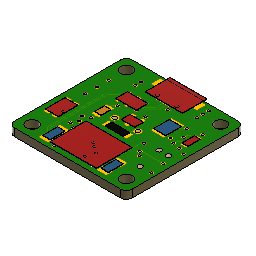
caps-lock-buzzer-v2-v5 (Autodesk Fusion 360 archive; units mm, degrees)
design "caps-lock-buzzer-v2-temp"
part number: 0.1uF 50V
part number: 1uF 16V X5R
part number: PIC16F1459-I/SS
part number: FMMT619TA
part number: 1N4148W-TP
part number: 2.2k
part number: CX-0905C
part number: PRTR5V0U2X
part number: RED
part number: KMR211NGLFS
Autodesk Fusion 360 part; units mm, degrees
sketch "sketch 305" plane through (0, 0, 0) normal (0, 0, 1) x (1, 0, 0)
  line L0 (1.27, 0) -> (24.13, 0)
  arc A0 (24.13, 0) -> (25.4, 1.27) centre (24.13, 1.27) ccw
  line L1 (25.4, 1.27) -> (25.4, 24.13)
  arc A1 (25.4, 24.13) -> (24.13, 25.4) centre (24.13, 24.13) ccw
  line L2 (24.13, 25.4) -> (1.27, 25.4)
  arc A2 (1.27, 25.4) -> (0, 24.13) centre (1.27, 24.13) ccw
  line L3 (0, 24.13) -> (0, 1.27)
  arc A3 (0, 1.27) -> (1.27, 0) centre (1.27, 1.27) ccw
  circle A4 centre (2.54, 2.54) radius 1.27
  circle A5 centre (2.54, 22.86) radius 1.27
  circle A6 centre (22.86, 22.86) radius 1.27
  circle A7 centre (22.86, 2.54) radius 1.27
extrude "Board" add sketch "sketch 305" along normal blind 1.6711 makes body 1 in component "Board"
sketch "sketch 829" plane through (0, 0, 0) normal (0, 0, 1) x (1, 0, 0)
  line L0 (-1.6, -0.8) -> (1.6, -0.8)
  line L1 (1.6, -0.8) -> (1.6, 0.8)
  line L2 (1.6, 0.8) -> (-1.6, 0.8)
  line L3 (-1.6, 0.8) -> (-1.6, -0.8)
extrude "C1206K" add sketch "sketch 829" along normal blind 0.1 separate body makes body 2 in component "C1206K"
sketch "sketch 961" plane through (0, 0, 0) normal (0, 0, 1) x (1, 0, 0)
  line L0 (-1.702, -1.304) -> (1.702, -1.304)
  line L1 (1.702, -1.304) -> (1.702, 1.304)
  line L2 (1.702, 1.304) -> (-1.702, 1.304)
  line L3 (-1.702, 1.304) -> (-1.702, -1.304)
extrude "C1210" add sketch "sketch 961" along normal blind 0.1 separate body makes body 3 in component "C1210"
sketch "sketch 1093" plane through (0, 0, 0) normal (0, 0, 1) x (1, 0, 0)
  line L0 (-4, -2.15) -> (4, -2.15)
  line L1 (4, -2.15) -> (4, 3.15)
  line L2 (4, 3.15) -> (-4, 3.15)
  line L3 (-4, 3.15) -> (-4, -2.15)
extrude "629105136821" add sketch "sketch 1093" along normal blind 0.1 separate body makes body 4 in component "629105136821"
sketch "sketch 1225" plane through (0, 0, 0) normal (0, 0, 1) x (1, 0, 0)
  line L0 (-4.966, -3.861) -> (4.966, -3.861)
  line L1 (4.966, -3.861) -> (4.966, 3.861)
  line L2 (4.966, 3.861) -> (-4.966, 3.861)
  line L3 (-4.966, 3.861) -> (-4.966, -3.861)
extrude "SSOP20_MC" add sketch "sketch 1225" along normal blind 0.1 separate body makes body 5 in component "SSOP20_MC"
sketch "sketch 1357" plane through (0, 0, 0) normal (0, 0, 1) x (1, 0, 0)
  line L0 (-1.422, -0.94) -> (1.473, -0.94)
  line L1 (1.473, -0.94) -> (1.473, 0.94)
  line L2 (1.473, 0.94) -> (-1.422, 0.94)
  line L3 (-1.422, 0.94) -> (-1.422, -0.94)
extrude "SOT-23" add sketch "sketch 1357" along normal blind 0.1 separate body makes body 6 in component "SOT-23"
sketch "sketch 1489" plane through (0, 0, 0) normal (0, 0, 1) x (1, 0, 0)
  line L0 (-1.95, -0.7) -> (1.95, -0.7)
  line L1 (1.95, -0.7) -> (1.95, 0.7)
  line L2 (1.95, 0.7) -> (-1.95, 0.7)
  line L3 (-1.95, 0.7) -> (-1.95, -0.7)
extrude "SOD123" add sketch "sketch 1489" along normal blind 0.1 separate body makes body 7 in component "SOD123"
sketch "sketch 1629" plane through (0, 0, 0) normal (0, 0, 1) x (1, 0, 0)
  line L0 (-1.067, -0.698) -> (1.056, -0.698)
  line L1 (1.056, -0.698) -> (1.056, 0.702)
  line L2 (1.056, 0.702) -> (-1.067, 0.702)
  line L3 (-1.067, 0.702) -> (-1.067, -0.698)
extrude "R0805" add sketch "sketch 1629" along normal blind 0.1 separate body makes body 8 in component "R0805"
sketch "sketch 1761" plane through (0, 0, 0) normal (0, 0, 1) x (1, 0, 0)
  line L0 (-4.8, -4.8) -> (4.8, -4.8)
  line L1 (4.8, -4.8) -> (4.8, 4.8)
  line L2 (4.8, 4.8) -> (-4.8, 4.8)
  line L3 (-4.8, 4.8) -> (-4.8, -4.8)
extrude "CUI_CX-0905C" add sketch "sketch 1761" along normal blind 0.1 separate body makes body 9 in component "CUI_CX-0905C"
sketch "sketch 1893" plane through (0, 0, 0) normal (0, 0, 1) x (1, 0, 0)
  line L0 (-0.4955, -1.5115) -> (5.5755, -1.5115)
  line L1 (5.5755, -1.5115) -> (5.5755, 1.5115)
  line L2 (5.5755, 1.5115) -> (-0.4955, 1.5115)
  line L3 (-0.4955, 1.5115) -> (-0.4955, -1.5115)
extrude "TC2030-MCP-NL" add sketch "sketch 1893" along normal blind 0.1 separate body makes body 10 in component "TC2030-MCP-NL"
sketch "sketch 2025" plane through (0, 0, 0) normal (0, 0, 1) x (1, 0, 0)
  line L0 (-2.896, -1.245) -> (1.499, -1.245)
  line L1 (1.499, -1.245) -> (1.499, 1.245)
  line L2 (1.499, 1.245) -> (-2.896, 1.245)
  line L3 (-2.896, 1.245) -> (-2.896, -1.245)
extrude "SOT143B" add sketch "sketch 2025" along normal blind 0.1 separate body makes body 11 in component "SOT143B"
sketch "sketch 2157" plane through (0, 0, 0) normal (0, 0, 1) x (1, 0, 0)
  line L0 (-0.625, -1.3334) -> (0.625, -1.3334)
  line L1 (0.625, -1.3334) -> (0.625, 1.3334)
  line L2 (0.625, 1.3334) -> (-0.625, 1.3334)
  line L3 (-0.625, 1.3334) -> (-0.625, -1.3334)
extrude "CHIPLED_0805_NOOUTLINE" add sketch "sketch 2157" along normal blind 0.1 separate body makes body 12 in component "CHIPLED_0805_NOOUTLINE"
sketch "sketch 2289" plane through (0, 0, 0) normal (0, 0, 1) x (1, 0, 0)
  line L0 (-2.1, -1.4) -> (2.1, -1.4)
  line L1 (2.1, -1.4) -> (2.1, 1.4)
  line L2 (2.1, 1.4) -> (-2.1, 1.4)
  line L3 (-2.1, 1.4) -> (-2.1, -1.4)
extrude "KMR2" add sketch "sketch 2289" along normal blind 0.1 separate body makes body 13 in component "KMR2"
sketch "sketch 457" plane through (0, 0, 0) normal (0, 0, 1) x (1, 0, 0)
  circle A0 centre (20.002, 8.255) radius 0.25
  circle A1 centre (2.54, 19.05) radius 0.25
  circle A2 centre (2.54, 16.51) radius 0.25
  circle A3 centre (2.54, 13.97) radius 0.25
  circle A4 centre (6.35, 22.225) radius 0.25
  circle A5 centre (6.35, 20.955) radius 0.25
  circle A6 centre (19.05, 24.13) radius 0.25
  circle A7 centre (19.05, 22.86) radius 0.25
  circle A8 centre (19.05, 21.59) radius 0.25
  circle A9 centre (22.86, 19.05) radius 0.25
  circle A10 centre (22.86, 13.97) radius 0.25
  circle A11 centre (24.448, 13.335) radius 0.25
  circle A12 centre (24.448, 6.35) radius 0.25
  circle A13 centre (8.89, 0.952) radius 0.25
  circle A14 centre (6.35, 9.525) radius 0.25
  circle A15 centre (6.35, 6.985) radius 0.25
  circle A16 centre (20.002, 14.922) radius 0.25
  circle A17 centre (14.199, 2.235) radius 0.25
  circle A18 centre (14.427, 19.914) radius 0.25
  circle A19 centre (11.112, 16.51) radius 0.25
  circle A20 centre (20.002, 18.415) radius 0.25
  circle A21 centre (14.808, 4.064) radius 0.25
  circle A22 centre (13.386, 5.08) radius 0.25
  circle A23 centre (19.164, 9.144) radius 0.25
  circle A24 centre (23.978, 9.347) radius 0.25
  circle A25 centre (12.573, 5.69) radius 0.25
  circle A26 centre (7.62, 6.35) radius 0.25
  circle A27 centre (7.622, 10.158) radius 0.25
  circle A28 centre (8.255, 15.24) radius 0.25
  circle A29 centre (13.335, 16.192) radius 0.25
  circle A30 centre (21.272, 16.51) radius 0.25
  circle A31 centre (18.098, 11.112) radius 0.25
  circle A32 centre (21.272, 14.288) radius 0.25
  circle A33 centre (3.492, 8.255) radius 0.25
  circle A34 centre (6.985, 8.255) radius 0.25
  circle A35 centre (14.775, 21.5) radius 0.35
  circle A36 centre (10.625, 21.5) radius 0.35
  circle A37 centre (15.2, 12.7) radius 0.45
  circle A38 centre (10.2, 12.7) radius 0.45
  circle A39 centre (22.047, 6.35) radius 0.4955
  circle A40 centre (21.031, 11.43) radius 0.4955
  circle A41 centre (23.063, 11.43) radius 0.4955
extrude "Extrude2" cut sketch "sketch 457" along normal blind 1.6711 bodies 1 in component "Board"
component "PCB Component" placed x (1, 0, 0) y (0, 1, 0) z (0, 0, 1) at (0, 0, 0)
component "Board" placed x (1, 0, 0) y (0, 1, 0) z (0, 0, 1) at (0, 0, 0) in component "PCB Component"
component "C1206K" placed x (0, -1, 0) y (1, 0, 0) z (0, 0, 1) at (6.579, 3.175, 1.6711) in component "PCB Component"
component "C1206K" placed x (0, 1, 0) y (-1, 0, 0) z (0, 0, 1) at (18.974, 3.34, 1.6711) in component "PCB Component"
component "C1210" placed x (0, -1, 0) y (1, 0, 0) z (0, 0, 1) at (17.78, 16.51, 1.6711) in component "PCB Component"
component "629105136821" placed x (-1, 0, 0) y (0, -1, 0) z (0, 0, 1) at (12.7, 23.95, 1.6711) in component "PCB Component"
component "SSOP20_MC" placed x (-1, 0, 0) y (0, -1, 0) z (0, 0, 1) at (12.725, 5.08, 1.6711) in component "PCB Component"
component "SOT-23" placed x (1, 0, 0) y (0, 1, 0) z (0, 0, 1) at (12.7, 13.97, 1.6711) in component "PCB Component"
component "SOD123" placed x (-1, 0, 0) y (0, -1, 0) z (0, 0, 1) at (12.7, 10.795, 1.6711) in component "PCB Component"
component "R0805" placed x (0, 1, 0) y (-1, 0, 0) z (0, 0, 1) at (7.62, 12.7, 1.6711) in component "PCB Component"
component "R0805" placed x (0, -1, 0) y (-1, 0, 0) z (0, 0, -1) at (22.86, 16.51, 0) in component "PCB Component"
component "CUI_CX-0905C" placed x (-1, 0, 0) y (0, 1, 0) z (0, 0, -1) at (12.7, 12.7, 0) in component "PCB Component"
component "TC2030-MCP-NL" placed x (0, 1, 0) y (1, 0, 0) z (0, 0, -1) at (22.047, 6.35, 0) in component "PCB Component"
component "SOT143B" placed x (-1, 0, 0) y (0, -1, 0) z (0, 0, 1) at (8.255, 17.621, 1.6711) in component "PCB Component"
component "CHIPLED_0805_NOOUTLINE" placed x (-1, 0, 0) y (0, -1, 0) z (0, 0, 1) at (22.86, 16.51, 1.6711) in component "PCB Component"
component "KMR2" placed x (0, -1, 0) y (1, 0, 0) z (0, 0, 1) at (2.54, 8.89, 1.6711) in component "PCB Component"
named bodies: "Board", "C1206K", "C1210", "629105136821", "SSOP20_MC", "SOT-23", "SOD123", "R0805", "CUI_CX-0905C", "TC2030-MCP-NL", "SOT143B", "CHIPLED_0805_NOOUTLINE", "KMR2"
